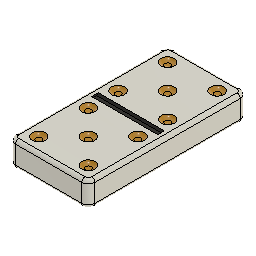
domino_v1 (Autodesk Fusion 360 design; units mm, degrees)
Autodesk Fusion 360 part; units mm, degrees
sketch "Sketch1" plane through (0, 0, 0) normal (0, 0, 1) x (1, 0, 0)
  line L0 (0, 0) -> (24, 0)
  line L1 (24, 0) -> (24, 48)
  line L2 (24, 48) -> (0, 48)
  line L3 (0, 48) -> (0, 0)
  dimension "d1" = 24
  dimension "d2" = 48
  constraint horizontal L0
  constraint vertical L1
  constraint horizontal L2
  constraint vertical L3
  constraint coincident L0.start L3.end
  measures "d1" distance of L0.start L0.end
  measures "d2" distance of L0.start L2.end
extrude "Extrude1" add sketch "Sketch1" along normal blind 7.5
sketch "Sketch2" plane through (0, 0, 7.5) normal (0, 0, 1) x (-1, 0, 0)
  line L0 (0, -48) -> (0, 0)
  line L1 (0, 0) -> (-24, 0)
  line L2 (-24, 0) -> (-24, -48)
  line L3 (-24, -48) -> (0, -48)
  line L4 (0, -24) -> (-24, -24) construction
  line L5 (-12, -48) -> (-12, 0) construction
  line L6 (-22, -25) -> (-2, -25)
  line L7 (-2, -25) -> (-2, -23)
  line L8 (-2, -23) -> (-22, -23)
  line L9 (-22, -23) -> (-22, -25)
  line L10 (-22, -25) -> (-2, -23) construction
  line L11 (-2, -25) -> (-22, -23) construction
  circle A0 centre (-19.5, -19.5) radius 2
  circle A1 centre (-19.5, -4.5) radius 2
  circle A2 centre (-4.5, -19.5) radius 2
  circle A3 centre (-4.5, -4.5) radius 2
  circle A4 centre (-4.5, -28.5) radius 2
  circle A5 centre (-19.5, -28.5) radius 2
  circle A6 centre (-19.5, -43.5) radius 2
  circle A7 centre (-4.5, -43.5) radius 2
  circle A8 centre (-12, -12) radius 2
  circle A9 centre (-12, -36) radius 2
  point P0 (-12, -24)
  dimension "d5" = 4.5
  dimension "d6" = 4.5
  dimension "d7" = 4.5
  dimension "d8" = 4.5
  dimension "d9" = 7.5
  dimension "d10" = 7.5
  constraint midpoint L0 L4.start
  constraint midpoint L2 L4.end
  constraint midpoint L3 L5.start
  constraint midpoint L1 L5.end
  constraint horizontal L6
  constraint perpendicular L6 L7
  constraint parallel L6 L8
  constraint parallel L7 L9
  constraint coincident L10 P0
  constraint coincident L11 P0
  constraint midpoint L4 P0
  constraint symmetric L5 A0 A2
  constraint symmetric L5 A1 A3
  constraint symmetric L4 A0 A5
  constraint symmetric L4 A1 A6
  constraint symmetric L4 A2 A4
  constraint symmetric L4 A3 A7
  constraint coincident L5 A8.centre
  constraint coincident L5 A9.centre
  measures "d5" distance of L4 A0.centre
  measures "d6" distance of L1 A1.centre
  measures "d7" distance of L2 A1.centre
  measures "d8" distance of L2 A0.centre
  measures "d9" vertical distance of A6.centre A9.centre
  measures "d10" vertical distance of A1.centre A8.centre
extrude "Extrude2" cut sketch "Sketch2" against normal blind 0.5 contours L6 L7 L8 L9
chamfer "Chamfer3" distance 0.5 angle 45 2 edges at (12, 23, 7) (12, 25, 7)
hole "Hole1" at (12, 36, 7.5) at (4.5, 43.5, 7.5) at (19.5, 43.5, 7.5) at (19.5, 28.5, 7.5) at (4.5, 28.5, 7.5) at (19.5, 19.5, 7.5) at (4.5, 19.5, 7.5) at (12, 12, 7.5) at (4.5, 4.5, 7.5) at (19.5, 4.5, 7.5) direction (0, 0, -1) diameter 4 depth 0.5 tip angle 150
fillet "Fillet1" radius 2 1 faces at (5.6403, 5.558, 6.8809)
fillet "Fillet1" radius 2 9 faces at (20.2778, 5.8472, 6.8809) (11.8838, 10.4488, 6.8809) (5.9015, 18.8251, 6.8809) (18.0136, 19.9585, 6.8809) (18.0136, 28.9585, 6.8809) (5.9015, 27.8251, 6.8809) (10.4444, 36, 6.8809) (20.6403, 42.442, 6.8809) (2.9444, 43.5, 6.8809)
fillet "Fillet2" radius 2 4 edges at (24, 0, 3.75) (0, 0, 3.75) (24, 48, 3.75) (0, 48, 3.75)
fillet "Fillet2" radius 1 8 edges at (24, 24, 7.5) (24, 24, 0) (12, 48, 7.5) (12, 48, 0) (0, 24, 7.5) (0, 24, 0) (12, 0, 7.5) (12, 0, 0)
